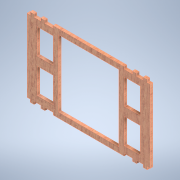
# Autodesk Inventor part: DoorFrameFront_V2
Saved by Autodesk Inventor 2022.2 (Build 262287000, 287)
## iProperties
Created: 2023-03-04
Part Number: DoorFrameFront_V2
Material: Wood (Oak)
Document SubType Name: Modeling
Designer: jaege
Density: 0.76 g/cm^3
Appearance: Red Oak - Natural Low Gloss
Author: jaege
Autodesk Inventor part; units mm, degrees
ref_plane "YZ Plane" through (0, 0, 0) normal (1, 0, 0) x (0, 1, 0)
ref_plane "XZ Plane" through (0, 0, 0) normal (0, 1, 0) x (-1, 0, 0)
ref_plane "XY Plane" through (0, 0, 0) normal (0, 0, 1) x (1, 0, 0)
sketch "Sketch1" plane through (0, 0, 0) normal (0, 0, 1) x (1, 0, 0)
  line L0 (45, -50) -> (-45, -50)
  line L1 (-45, -50) -> (-45, 50)
  line L2 (-45, 50) -> (45, 50)
  line L3 (45, 50) -> (45, -50)
  line L4 (45, -50) -> (-45, 50) construction
  line L5 (-45, -50) -> (45, 50) construction
  line L6 (53, 58) -> (-53, 58)
  line L7 (-53, 58) -> (-53, 54.5)
  line L8 (-53, -58) -> (53, -58)
  line L9 (53, -58) -> (53, -54.5)
  line L10 (-20, 50) -> (20, 50)
  line L11 (-20, -50) -> (20, -50)
  line L12 (-45, -20) -> (-45, 20)
  line L13 (45, -20) -> (45, 20)
  line L14 (-53, 6.5) -> (-77, 6.5)
  line L15 (-53, -6.5) -> (-53, 6.5) construction
  line L16 (-53, 0) -> (53, 0)
  line L17 (0, 50) -> (0, -50)
  line L18 (-53, 6.5) -> (-53, -6.5) construction
  line L19 (-53, -6.5) -> (-53, -44.5)
  line L20 (53, 6.5) -> (53, 44.5)
  line L21 (53, -6.5) -> (53, 6.5) construction
  line L22 (-92, -6.5) -> (-77, -6.5) construction
  line L23 (-77, -6.5) -> (-77, -44.5)
  line L24 (-77, -58) -> (-92, -58) construction
  line L25 (-92, -58) -> (-92, -54.5) construction
  line L26 (-92, -58) -> (-77, -58) construction
  line L27 (-77, -58) -> (-77, -58.5) construction
  line L28 (-77, -58.5) -> (-81.5, -58.5) construction
  line L29 (-92, -58.5) -> (-92, -58) construction
  line L30 (-92, -54.5) -> (-87.5, -54.5)
  line L31 (-87.5, -54.5) -> (-87.5, -58.5)
  line L32 (-81.5, -58.5) -> (-81.5, -54.5)
  line L33 (-81.5, -54.5) -> (-77, -54.5)
  line L34 (-77, 6.5) -> (-77, 44.5)
  line L35 (-77, 58) -> (-92, 58) construction
  line L36 (-92, 58) -> (-92, 54.5) construction
  line L37 (-92, 58) -> (-77, 58) construction
  line L38 (-77, 58) -> (-77, 58.5) construction
  line L39 (-77, 58.5) -> (-81.5, 58.5) construction
  line L40 (-92, 58.5) -> (-92, 58) construction
  line L41 (-92, 54.5) -> (-87.5, 54.5)
  line L42 (-87.5, 54.5) -> (-87.5, 58.5)
  line L43 (-81.5, 58.5) -> (-81.5, 54.5)
  line L44 (-81.5, 54.5) -> (-77, 54.5)
  line L45 (-77, 6.5) -> (-92, 6.5) construction
  line L46 (-92, -6.5) -> (-77, -6.5) construction
  line L47 (-77, -6.5) -> (-53, -6.5)
  line L48 (-77, 54.5) -> (-77, 58) construction
  line L49 (-92, 54.5) -> (-92, 6.5)
  line L50 (-87.5, 58.5) -> (-92, 58.5) construction
  line L51 (-81.5, 58.5) -> (-87.5, 58.5)
  line L52 (-92, -54.5) -> (-92, -6.5)
  line L53 (-87.5, -58.5) -> (-92, -58.5) construction
  line L54 (-81.5, -58.5) -> (-87.5, -58.5)
  line L55 (-77, -54.5) -> (-77, -58) construction
  line L56 (-77, 54.5) -> (-71.5, 54.5)
  line L57 (-53, 54.5) -> (-53, 44.5) construction
  line L58 (-53, 44.5) -> (-77, 44.5)
  line L59 (-77, 44.5) -> (-77, 54.5) construction
  line L60 (-77, -54.5) -> (-71.5, -54.5)
  line L61 (-53, -54.5) -> (-53, -54)
  line L62 (-53, -44.5) -> (-77, -44.5)
  line L63 (-77, -44.5) -> (-77, -54.5) construction
  line L64 (-71.5, 54.5) -> (-65.5, 54.5) construction
  line L65 (-65.5, 54.5) -> (-65.5, 58.5)
  line L66 (-65.5, 58.5) -> (-71.5, 58.5)
  line L67 (-71.5, 58.5) -> (-71.5, 54.5)
  line L68 (-71.5, -54.5) -> (-65.5, -54.5) construction
  line L69 (-65.5, -54.5) -> (-65.5, -58.5)
  line L70 (-65.5, -58.5) -> (-71.5, -58.5)
  line L71 (-71.5, -58.5) -> (-71.5, -54.5)
  line L72 (-71.5, 54.5) -> (-65.5, 54.5) construction
  line L73 (-65.5, 54.5) -> (-53, 54.5)
  line L74 (-77, 44.5) -> (-77, 54.5) construction
  line L75 (-53, 44.5) -> (-53, 6.5)
  line L76 (-53, 54.5) -> (-53, 44.5) construction
  line L77 (-77, -44.5) -> (-77, -54.5) construction
  line L78 (-53, -44.5) -> (-53, -54.5) construction
  line L79 (-53, -54) -> (-53, -44.5) construction
  line L80 (-65.5, -54.5) -> (-53, -54.5)
  line L81 (-71.5, -54.5) -> (-65.5, -54.5) construction
  line L82 (-53, -54.5) -> (-53, -58)
  line L83 (53, 6.5) -> (77, 6.5)
  line L84 (92, -6.5) -> (77, -6.5) construction
  line L85 (77, -6.5) -> (77, -44.5)
  line L86 (77, -58) -> (92, -58) construction
  line L87 (92, -58) -> (92, -54.5) construction
  line L88 (92, -58) -> (77, -58) construction
  line L89 (77, -58) -> (77, -58.5) construction
  line L90 (77, -58.5) -> (81.5, -58.5) construction
  line L91 (92, -58.5) -> (92, -58) construction
  line L92 (92, -54.5) -> (87.5, -54.5)
  line L93 (87.5, -54.5) -> (87.5, -58.5)
  line L94 (81.5, -58.5) -> (81.5, -54.5)
  line L95 (81.5, -54.5) -> (77, -54.5)
  line L96 (92, 54.5) -> (87.5, 54.5)
  line L97 (92, 58) -> (92, 54.5) construction
  line L98 (77, 6.5) -> (77, 44.5)
  line L99 (81.5, 54.5) -> (77, 54.5)
  line L100 (77, 58) -> (92, 58) construction
  line L101 (92, 58) -> (77, 58) construction
  line L102 (77, 58) -> (77, 58.5) construction
  line L103 (77, 58.5) -> (81.5, 58.5) construction
  line L104 (81.5, 58.5) -> (81.5, 54.5)
  line L105 (92, 58.5) -> (92, 58) construction
  line L106 (87.5, 54.5) -> (87.5, 58.5)
  line L107 (77, 6.5) -> (92, 6.5) construction
  line L108 (92, -6.5) -> (77, -6.5) construction
  line L109 (77, -6.5) -> (53, -6.5)
  line L110 (77, 54.5) -> (77, 58) construction
  line L111 (92, 54.5) -> (92, 6.5)
  line L112 (87.5, 58.5) -> (92, 58.5) construction
  line L113 (81.5, 58.5) -> (87.5, 58.5)
  line L114 (92, -54.5) -> (92, -6.5)
  line L115 (87.5, -58.5) -> (92, -58.5) construction
  line L116 (81.5, -58.5) -> (87.5, -58.5)
  line L117 (77, -54.5) -> (77, -58) construction
  line L118 (77, 54.5) -> (71.5, 54.5)
  line L119 (53, 44.5) -> (77, 44.5)
  line L120 (77, 44.5) -> (77, 54.5) construction
  line L121 (77, -54.5) -> (71.5, -54.5)
  line L122 (53, -44.5) -> (77, -44.5)
  line L123 (77, -44.5) -> (77, -54.5) construction
  line L124 (71.5, 54.5) -> (65.5, 54.5) construction
  line L125 (65.5, 54.5) -> (65.5, 58.5)
  line L126 (65.5, 58.5) -> (71.5, 58.5)
  line L127 (71.5, 58.5) -> (71.5, 54.5)
  line L128 (71.5, -54.5) -> (65.5, -54.5) construction
  line L129 (65.5, -54.5) -> (65.5, -58.5)
  line L130 (65.5, -58.5) -> (71.5, -58.5)
  line L131 (71.5, -58.5) -> (71.5, -54.5)
  line L132 (71.5, 54.5) -> (65.5, 54.5) construction
  line L133 (65.5, 54.5) -> (53, 54.5)
  line L134 (77, 44.5) -> (77, 54.5) construction
  line L135 (77, -44.5) -> (77, -54.5) construction
  line L136 (65.5, -54.5) -> (53, -54.5)
  line L137 (71.5, -54.5) -> (65.5, -54.5) construction
  line L138 (53, 44.5) -> (53, 54.5) construction
  line L139 (53, 54.5) -> (53, 58)
  line L140 (53, -44.5) -> (53, -6.5)
  line L141 (53, -54.5) -> (53, -44.5) construction
  line L142 (-92, 6.5) -> (-92, -6.5)
  line L143 (92, 6.5) -> (92, -6.5)
  point P0 (0, 0)
  point P1 (0, 54)
  point P2 (0, 0)
  point P3 (-49, 0)
  point P4 (0, 0)
  point P5 (-53, 0)
  point P6 (0, 0)
  point P7 (0, 0)
  point P8 (-84.5, -58)
  point P9 (-84.5, 58)
  point P10 (-65, 44.5)
  point P11 (-81.5, 56.5)
  point P12 (-71.5, 56.5)
  point P13 (84.5, -58)
  point P14 (84.5, 58)
  point P15 (65, 44.5)
  point P16 (81.5, 56.5)
  point P17 (71.5, 56.5)
  dimension "d0" = 100
  dimension "d1" = 90
  dimension "d2" = 8
  dimension "d16" = 15
  dimension "d17" = 0.5
  dimension "d18" = 6
  dimension "d19" = 4.5
  dimension "d20" = 4.5
  dimension "d21" = 4
  dimension "d24" = 10
  dimension "d25" = 10
  dimension "d27" = 10
  dimension "d28" = 6
  dimension "d29" = 8
  dimension "d30" = 8
  dimension "d31" = 4.5
  dimension "d32" = 24
  constraints: 288 end point, 82 parallel, 58 symmetric about line, 27 perpendicular, 15 horizontal, 14 midpoint, 12 point on line, 4 horizontal alignment, 3 vertical alignment, 1 collinear
  measures "d0" distance of L0.end L1.end
  measures "d1" distance of L1.end L2.end
  measures "d2" distance between parallel lines of L2 L6
  measures "d16" distance of L24.start L24.end
  measures "d17" distance of L24.start L27.end
  measures "d18" distance between parallel lines of L32 L31
  measures "d19" distance of L32.end L33.end
  measures "d20" distance of L25.end L30.end
  measures "d21" distance of L30.end L31.end
  measures "d24" distance from line of point (-65, 44.5) L56
  measures "d25" distance between parallel lines of L62 L60
  measures "d27" distance of L70.end L28.end
  measures "d28" distance of L69.end L70.end
  measures "d29" distance between parallel lines of L1 L19
  measures "d30" distance between parallel lines of L3 L20
  measures "d31" distance between parallel lines of L2 L73
  measures "d32" distance between parallel lines of L75 L34
extrude "Extrusion1" add sketch "Sketch1" along normal blind 4
body "Solid1"
